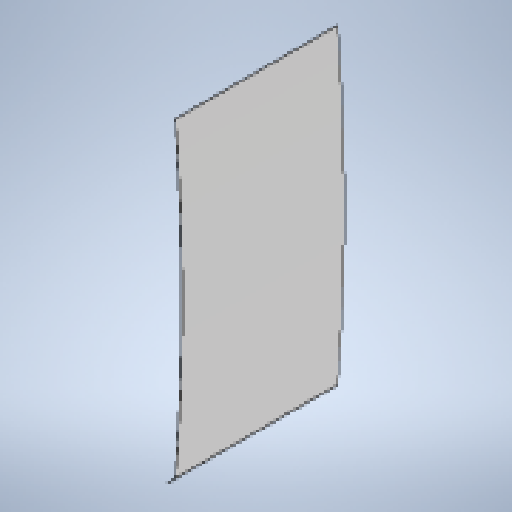
# Autodesk Inventor part: MSC 302 sheet board main
Saved by Autodesk Inventor 2025 (Build 290162010, 162A)
## iProperties
Created: 2024-04-18
Part Number: MSC 302 sheet board main
Material: AISI304
Document SubType Name: Sheet Metal
Designer: admin
Stock Number: МОО 302 лист борт основной
Density: 8 g/cm^3
Flat Pattern Width: 98 cm
Flat Pattern Length: 194.828 cm
Flat Pattern Area: 19093.2 cm^2
Sheet Metal Rule: AISI304 3mm
Sheet Metal Width: 980,000 mm
Sheet Metal Length: 1948,285 mm
Sheet Metal Area: 1909318,912 mm^2
Appearance: Default
Mass: 45827.4 g
Surface Area: 38365.2 cm^2
Volume: 5728.43 cm^3
Author: admin
Autodesk Inventor part; units mm, degrees
ref_plane "YZ Plane" through (0, 0, 0) normal (1, 0, 0) x (0, 1, 0)
ref_plane "XZ Plane" through (0, 0, 0) normal (0, 1, 0) x (-1, 0, 0)
ref_plane "XY Plane" through (0, 0, 0) normal (0, 0, 1) x (1, 0, 0)
sketch "Sketch1" plane through (0, 0, 0) normal (0, 0, 1) x (1, 0, 0)
  line L0 (0, 100) -> (0, 50) construction
  line L1 (0, 47) -> (0, 0) construction
  arc A0 (0.159434, 1.869277) -> (0, 1880) centre (-11009.945504, 940) ccw
  arc A1 (0, 0) -> (0.159434, 1.869277) centre (-11009.945504, 940) ccw construction
  arc A2 (-1.349222, -1.302929) -> (0.159434, 1.869277) centre (-4.822514, 2.29377) ccw
  line L2 (-1.349222, -1.302929) -> (0, 0) construction
  line L3 (-46.757087, -45.152794) -> (-1.349222, -1.302929)
  line L4 (-41.190716, -50.91694) -> (-46.757087, -45.152794) construction
  line L5 (0, 0) -> (0, 1880) construction
  line L6 (0, 0) -> (1.875639, 0) construction
  dimension "d121" = 5
  dimension "d122" = 65
  dimension "d123" = 11050
  dimension "d124" = 136
  dimension "d125" = 1880
  measures "d121" radius of A2
  measures "d122" distance of L1.end L3.start
  measures "d123" radius of A0
  measures "d124" angle of L2 L6
  measures "d125" distance of L1.end L5.end
contour flange "Contour Flange2" sketch "Sketch1" thickness 3 bend radius 5 width 980 along (0, 0, 1) mid plane no both sides no wall seen from (-24.053155, -23.227861, 0) lies toward (0.6946584, -0.7193398, 0) curves L3 A2 A0
bend "Bend2"
corner "Corner2"
sketch "Sketch4" plane through (-1.349222, -1.302929, 980) normal (-0.6946584, 0.7193398, 0) x (0.7193398, 0.6946584, 0)
  line L0 (-51.124361, 36.175726) -> (-51.124361, 160.841262) construction
  line L1 (-51.124361, 160.841262) -> (-39.124361, 160.841262) construction
  line L2 (-39.124361, 160.841262) -> (-39.124361, 36.175726) construction
  line L3 (-39.124361, 36.175726) -> (-51.124361, 36.175726) construction
  line L4 (-63.124361, 0) -> (-63.124361, 980)
  point P0 (1.875639, 980)
  dimension "d127" = 12
  dimension "d128" = 12
  constraints: 2 other
  measures "d127" distance between parallel lines of L0 L4
  measures "d128" distance of L0.end L1.end
mark "Mark2"
equation "\"d36\" = Thickness"
equation "\"d37\" = BendReliefWidth"
equation "\"d38\" = BendReliefDepth"
equation "\"d39\" = MinimumRemnant"
equation "\"d40\" = TransitionRadius"
equation "\"d42\" = BendRadius"
equation "\"d44\" = CornerReliefSize"
equation "\"d45\" = GapSize"
equation "\"d46\" = JacobiRadiusSize"
equation "\"BendReliefWidth\" = Thickness"
equation "\"BendReliefDepth\" = 0.5 * Thickness"
equation "\"CornerReliefSize\" = 4 * Thickness"
equation "\"MinimumRemnant\" = 2 * Thickness"
equation "\"GapSize\" = Thickness"
equation "\"Thickness\" = 3"
equation "\"TransitionRadius\" = 5"
equation "\"BendRadius\" = 5"
equation "\"JacobiRadiusSize\" = 5"
body "Solid3"
